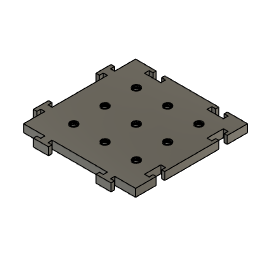
Threaded Optical Breadboard (Autodesk Fusion 360 design; units mm, degrees)
Autodesk Fusion 360 part; units mm, degrees
(part 1 of 2)
sketch "Sketch1" plane through (0, 0, 0) normal (0, 0, 1) x (1, 0, 0) in component "Breadboard"
  line L0 (20.188, 20.188) -> (-20.188, 20.188) construction
  line L1 (-20.188, 20.188) -> (-20.188, -20.188) construction
  line L2 (-20.188, -20.188) -> (20.188, -20.188) construction
  line L3 (20.188, -20.188) -> (20.188, 20.188) construction
  line L4 (20.188, 20.188) -> (-20.188, -20.188) construction
  line L5 (-20.188, 20.188) -> (20.188, -20.188) construction
  line L6 (-20.188, 20.188) -> (20.188, 20.188) construction
  line L7 (20.188, 20.188) -> (20.188, 60.564) construction
  line L8 (20.188, 60.564) -> (-20.188, 60.564) construction
  line L9 (-20.188, 60.564) -> (-20.188, 20.188) construction
  line L10 (20.188, 60.564) -> (60.564, 60.564) construction
  line L11 (60.564, 60.564) -> (60.564, 20.188) construction
  line L12 (60.564, 20.188) -> (20.188, 20.188) construction
  line L13 (20.188, 20.188) -> (20.188, 60.564) construction
  line L14 (60.564, 20.188) -> (20.188, 20.188) construction
  line L15 (20.188, 20.188) -> (20.188, -20.188) construction
  line L16 (20.188, -20.188) -> (60.564, -20.188) construction
  line L17 (60.564, -20.188) -> (60.564, 20.188) construction
  line L18 (-20.188, -20.188) -> (20.188, -20.188) construction
  line L19 (20.188, -20.188) -> (20.188, -60.564) construction
  line L20 (20.188, -60.564) -> (-20.188, -60.564) construction
  line L21 (-20.188, -60.564) -> (-20.188, -20.188) construction
  line L22 (20.188, -20.188) -> (60.564, -20.188) construction
  line L23 (60.564, -20.188) -> (60.564, -60.564) construction
  line L24 (60.564, -60.564) -> (20.188, -60.564) construction
  line L25 (20.188, -60.564) -> (20.188, -20.188) construction
  line L26 (-20.188, 20.188) -> (-60.564, 20.188) construction
  line L27 (-60.564, 20.188) -> (-60.564, 60.564) construction
  line L28 (-60.564, 60.564) -> (-20.188, 60.564) construction
  line L29 (-20.188, 60.564) -> (-20.188, 20.188) construction
  line L30 (-60.564, 20.188) -> (-20.188, 20.188) construction
  line L31 (-20.188, 20.188) -> (-20.188, -20.188) construction
  line L32 (-20.188, -20.188) -> (-60.564, -20.188) construction
  line L33 (-60.564, -20.188) -> (-60.564, 20.188) construction
  line L34 (-60.564, -20.188) -> (-20.188, -20.188) construction
  line L35 (-20.188, -20.188) -> (-20.188, -60.564) construction
  line L36 (-20.188, -60.564) -> (-60.564, -60.564) construction
  line L37 (-60.564, -60.564) -> (-60.564, -20.188) construction
  line L38 (72.5, 72.5) -> (-72.5, 72.5)
  line L39 (-72.5, 72.5) -> (-72.5, -72.5)
  line L40 (-72.5, -72.5) -> (72.5, -72.5)
  line L41 (72.5, -72.5) -> (72.5, 72.5)
  line L42 (72.5, 72.5) -> (-72.5, -72.5) construction
  line L43 (-72.5, 72.5) -> (72.5, -72.5) construction
  circle A0 centre (-40.376, 40.376) radius 5
  circle A1 centre (0, 40.376) radius 5
  circle A2 centre (40.376, 40.376) radius 5
  circle A3 centre (40.376, 0) radius 5
  circle A4 centre (0, 0) radius 5
  circle A5 centre (40.376, -40.376) radius 5
  circle A6 centre (0, -40.376) radius 5
  circle A7 centre (-40.376, -40.376) radius 5
  circle A8 centre (-40.376, 0) radius 5
  line L44 (-60.564, 60.564) -> (-60.564, 72.5) construction
  line L45 (-20.188, 60.564) -> (-20.188, 72.5) construction
  line L46 (20.188, 60.564) -> (20.188, 72.5) construction
  line L47 (60.564, 60.564) -> (60.564, 72.5) construction
  line L48 (60.564, 60.564) -> (72.5, 60.564) construction
  line L49 (60.564, 20.188) -> (72.5, 20.188) construction
  line L50 (60.564, -20.188) -> (72.5, -20.188) construction
  line L51 (60.564, -60.564) -> (72.5, -60.564) construction
  line L52 (60.564, -60.564) -> (60.564, -72.5) construction
  line L53 (20.188, -60.564) -> (20.188, -72.5) construction
  line L54 (-20.188, -60.564) -> (-20.188, -72.5) construction
  line L55 (-60.564, -60.564) -> (-60.564, -72.5) construction
  line L56 (-60.564, -60.564) -> (-72.5, -60.564) construction
  line L57 (-60.564, -20.188) -> (-72.5, -20.188) construction
  line L58 (-60.564, 20.188) -> (-72.5, 20.188) construction
  line L59 (-60.564, 60.564) -> (-72.5, 60.564) construction
  line L60 (-40.376, 60.564) -> (-40.376, 72.5) construction
  line L61 (40.376, 60.564) -> (40.376, 72.5) construction
  line L62 (60.564, 40.376) -> (72.5, 40.376) construction
  line L63 (60.564, -40.376) -> (72.5, -40.376) construction
  line L64 (40.376, -60.564) -> (40.376, -72.5) construction
  line L65 (-40.376, -60.564) -> (-40.376, -72.5) construction
  line L66 (-60.564, -40.376) -> (-72.5, -40.376) construction
  line L67 (-60.564, 40.376) -> (-72.5, 40.376) construction
  line L68 (-40.376, 72.5) -> (-45.376, 72.5) construction
  line L69 (-40.376, 72.5) -> (-35.376, 72.5) construction
  line L70 (-45.376, 72.5) -> (-35.376, 72.5)
  line L71 (-35.376, 72.5) -> (-35.376, 67.5)
  line L72 (-35.376, 67.5) -> (-45.376, 67.5)
  line L73 (-45.376, 67.5) -> (-45.376, 72.5)
  line L74 (-35.376, 67.5) -> (-30.376, 67.5)
  line L75 (-30.376, 67.5) -> (-30.376, 62.5)
  line L76 (-30.376, 62.5) -> (-35.376, 62.5)
  line L77 (-35.376, 62.5) -> (-35.376, 67.5)
  line L78 (-35.376, 62.5) -> (-45.376, 62.5)
  line L79 (-45.376, 62.5) -> (-45.376, 67.5)
  line L80 (-45.376, 67.5) -> (-35.376, 67.5)
  line L81 (-35.376, 67.5) -> (-35.376, 62.5)
  line L82 (-45.376, 67.5) -> (-50.376, 67.5)
  line L83 (-50.376, 67.5) -> (-50.376, 62.5)
  line L84 (-50.376, 62.5) -> (-45.376, 62.5)
  line L85 (-45.376, 62.5) -> (-45.376, 67.5)
  line L86 (40.376, 72.5) -> (35.376, 72.5) construction
  line L87 (40.376, 72.5) -> (45.376, 72.5) construction
  line L88 (35.376, 72.5) -> (45.376, 72.5)
  line L89 (45.376, 72.5) -> (45.376, 67.5)
  line L90 (45.376, 67.5) -> (35.376, 67.5)
  line L91 (35.376, 67.5) -> (35.376, 72.5)
  line L92 (35.376, 67.5) -> (45.376, 67.5)
  line L93 (45.376, 67.5) -> (45.376, 62.5)
  line L94 (45.376, 62.5) -> (35.376, 62.5)
  line L95 (35.376, 62.5) -> (35.376, 67.5)
  line L96 (45.376, 62.5) -> (50.376, 62.5)
  line L97 (50.376, 62.5) -> (50.376, 67.5)
  line L98 (50.376, 67.5) -> (45.376, 67.5)
  line L99 (45.376, 67.5) -> (45.376, 62.5)
  line L100 (35.376, 62.5) -> (30.376, 62.5)
  line L101 (30.376, 62.5) -> (30.376, 67.5)
  line L102 (30.376, 67.5) -> (35.376, 67.5)
  line L103 (35.376, 67.5) -> (35.376, 62.5)
  line L104 (72.5, 40.376) -> (72.5, 45.376) construction
  line L105 (72.5, 40.376) -> (72.5, 35.376) construction
  line L106 (72.5, 45.376) -> (67.5, 45.376)
  line L107 (67.5, 45.376) -> (67.5, 35.376)
  line L108 (67.5, 35.376) -> (72.5, 35.376)
  line L109 (72.5, 35.376) -> (72.5, 45.376)
  line L110 (67.5, 45.376) -> (62.5, 45.376)
  line L111 (62.5, 45.376) -> (62.5, 35.376)
  line L112 (62.5, 35.376) -> (67.5, 35.376)
  line L113 (67.5, 35.376) -> (67.5, 45.376)
  line L114 (67.5, 45.376) -> (62.5, 45.376)
  line L115 (62.5, 45.376) -> (62.5, 50.376)
  line L116 (62.5, 50.376) -> (67.5, 50.376)
  line L117 (67.5, 50.376) -> (67.5, 45.376)
  line L118 (67.5, 35.376) -> (62.5, 35.376)
  line L119 (62.5, 35.376) -> (62.5, 30.376)
  line L120 (62.5, 30.376) -> (67.5, 30.376)
  line L121 (67.5, 30.376) -> (67.5, 35.376)
  line L122 (72.5, -40.376) -> (72.5, -35.376) construction
  line L123 (72.5, -40.376) -> (72.5, -45.376) construction
  line L124 (72.5, -45.376) -> (67.5, -45.376)
  line L125 (67.5, -45.376) -> (67.5, -35.376)
  line L126 (67.5, -35.376) -> (72.5, -35.376)
  line L127 (72.5, -35.376) -> (72.5, -45.376)
  line L128 (67.5, -35.376) -> (62.5, -35.376)
  line L129 (62.5, -35.376) -> (62.5, -45.376)
  line L130 (62.5, -45.376) -> (67.5, -45.376)
  line L131 (67.5, -45.376) -> (67.5, -35.376)
  line L132 (67.5, -35.376) -> (62.5, -35.376)
  line L133 (62.5, -35.376) -> (62.5, -30.376)
  line L134 (62.5, -30.376) -> (67.5, -30.376)
  line L135 (67.5, -30.376) -> (67.5, -35.376)
  line L136 (67.5, -45.376) -> (62.5, -45.376)
  line L137 (62.5, -45.376) -> (62.5, -50.376)
  line L138 (62.5, -50.376) -> (67.5, -50.376)
  line L139 (67.5, -50.376) -> (67.5, -45.376)
  line L140 (40.376, -72.5) -> (45.376, -72.5)
  line L141 (40.376, -72.5) -> (35.376, -72.5)
  line L142 (-40.376, -72.5) -> (-35.376, -72.5)
  line L143 (-40.376, -72.5) -> (-45.376, -72.5)
  line L144 (-72.5, -40.376) -> (-72.5, -45.376)
  line L145 (-72.5, -40.376) -> (-72.5, -35.376)
  line L146 (-72.5, 40.376) -> (-72.5, 35.376)
  line L147 (-72.5, 40.376) -> (-72.5, 45.376)
  line L148 (-72.5, 45.376) -> (-77.5, 45.376)
  line L149 (-77.5, 45.376) -> (-77.5, 35.376)
  line L150 (-77.5, 35.376) -> (-72.5, 35.376)
  line L151 (-72.5, 35.376) -> (-72.5, 45.376)
  line L152 (-77.5, 35.376) -> (-82.5, 35.376)
  line L153 (-82.5, 35.376) -> (-82.5, 45.376)
  line L154 (-82.5, 45.376) -> (-77.5, 45.376)
  line L155 (-77.5, 45.376) -> (-77.5, 35.376)
  line L156 (-77.5, 35.376) -> (-82.5, 35.376)
  line L157 (-82.5, 35.376) -> (-82.5, 30.376)
  line L158 (-82.5, 30.376) -> (-77.5, 30.376)
  line L159 (-77.5, 30.376) -> (-77.5, 35.376)
  line L160 (-77.5, 45.376) -> (-82.5, 45.376)
  line L161 (-82.5, 45.376) -> (-82.5, 50.376)
  line L162 (-82.5, 50.376) -> (-77.5, 50.376)
  line L163 (-77.5, 50.376) -> (-77.5, 45.376)
  line L164 (-72.5, -35.376) -> (-77.5, -35.376)
  line L165 (-77.5, -35.376) -> (-77.5, -45.376)
  line L166 (-77.5, -45.376) -> (-72.5, -45.376)
  line L167 (-72.5, -45.376) -> (-72.5, -35.376)
  line L168 (-77.5, -45.376) -> (-82.5, -45.376)
  line L169 (-82.5, -45.376) -> (-82.5, -35.376)
  line L170 (-82.5, -35.376) -> (-77.5, -35.376)
  line L171 (-77.5, -35.376) -> (-77.5, -45.376)
  line L172 (-77.5, -35.376) -> (-82.5, -35.376)
  line L173 (-82.5, -35.376) -> (-82.5, -30.376)
  line L174 (-82.5, -30.376) -> (-77.5, -30.376)
  line L175 (-77.5, -30.376) -> (-77.5, -35.376)
  line L176 (-77.5, -45.376) -> (-82.5, -45.376)
  line L177 (-82.5, -45.376) -> (-82.5, -50.376)
  line L178 (-82.5, -50.376) -> (-77.5, -50.376)
  line L179 (-77.5, -50.376) -> (-77.5, -45.376)
  line L180 (-45.376, -72.5) -> (-35.376, -72.5)
  line L181 (-35.376, -72.5) -> (-35.376, -77.5)
  line L182 (-35.376, -77.5) -> (-45.376, -77.5)
  line L183 (-45.376, -77.5) -> (-45.376, -72.5)
  line L184 (-35.376, -77.5) -> (-45.376, -77.5)
  line L185 (-45.376, -77.5) -> (-45.376, -82.5)
  line L186 (-45.376, -82.5) -> (-35.376, -82.5)
  line L187 (-35.376, -82.5) -> (-35.376, -77.5)
  line L188 (-35.376, -82.5) -> (-30.376, -82.5)
  line L189 (-30.376, -82.5) -> (-30.376, -77.5)
  line L190 (-30.376, -77.5) -> (-35.376, -77.5)
  line L191 (-35.376, -77.5) -> (-35.376, -82.5)
  line L192 (-45.376, -82.5) -> (-50.376, -82.5)
  line L193 (-50.376, -82.5) -> (-50.376, -77.5)
  line L194 (-50.376, -77.5) -> (-45.376, -77.5)
  line L195 (-45.376, -77.5) -> (-45.376, -82.5)
  line L196 (45.376, -72.5) -> (35.376, -72.5)
  line L197 (35.376, -72.5) -> (35.376, -77.5)
  line L198 (35.376, -77.5) -> (45.376, -77.5)
  line L199 (45.376, -77.5) -> (45.376, -72.5)
  line L200 (35.376, -77.5) -> (45.376, -77.5)
  line L201 (45.376, -77.5) -> (45.376, -82.5)
  line L202 (45.376, -82.5) -> (35.376, -82.5)
  line L203 (35.376, -82.5) -> (35.376, -77.5)
  line L204 (45.376, -77.5) -> (50.376, -77.5)
  line L205 (50.376, -77.5) -> (50.376, -82.5)
  line L206 (50.376, -82.5) -> (45.376, -82.5)
  line L207 (45.376, -82.5) -> (45.376, -77.5)
  line L208 (35.376, -82.5) -> (30.376, -82.5)
  line L209 (30.376, -82.5) -> (30.376, -77.5)
  line L210 (30.376, -77.5) -> (35.376, -77.5)
  line L211 (35.376, -77.5) -> (35.376, -82.5)
  dimension "d3" = 40.376
  dimension "d4" = 40.376
  dimension "d5" = 40.376
  dimension "d6" = 40.376
  dimension "d7" = 40.376
  dimension "d8" = 40.376
  dimension "d9" = 40.376
  dimension "d10" = 40.376
  dimension "d11" = 145
  dimension "d12" = 145
  dimension "d13" = 10
  dimension "d14" = 10
  dimension "d15" = 10
  dimension "d16" = 10
  dimension "d17" = 10
  dimension "d18" = 10
  dimension "d19" = 10
  dimension "d20" = 10
  dimension "d21" = 10
  dimension "d22" = 5
  dimension "d23" = 5
  dimension "d24" = 10
  dimension "d25" = 5
  dimension "d26" = 5
  dimension "d27" = 5
  dimension "d28" = 5
  dimension "d29" = 5
  dimension "d30" = 5
  dimension "d31" = 5
  dimension "d32" = 5
  dimension "d33" = 5
  dimension "d34" = 5
  dimension "d35" = 5
  dimension "d36" = 5
  dimension "d37" = 5
  dimension "d38" = 5
  dimension "d39" = 5
  dimension "d40" = 5
  dimension "d41" = 5
  dimension "d42" = 5
  dimension "d43" = 5
  dimension "d44" = 5
  dimension "d45" = 5
  dimension "d46" = 5
  dimension "d47" = 5
  dimension "d48" = 5
  dimension "d49" = 5
  dimension "d50" = 5
  dimension "d51" = 5
  dimension "d52" = 5
  dimension "d53" = 5
  dimension "d54" = 5
  dimension "d55" = 5
  dimension "d56" = 5
  dimension "d57" = 5
  dimension "d58" = 5
  dimension "d59" = 5
  dimension "d60" = 5
  dimension "d61" = 5
  dimension "d62" = 5
  dimension "d63" = 5
  dimension "d64" = 5
  dimension "d65" = 5
  dimension "d66" = 5
  dimension "d67" = 10
  dimension "d68" = 5
  dimension "d69" = 5
  dimension "d70" = 5
  constraint coincident A4.centre origin
  constraint horizontal L0
  constraint perpendicular L0 L1
  constraint parallel L0 L2
  constraint parallel L1 L3
  constraint coincident L4 A4.centre
  constraint coincident L5 A4.centre
  constraint horizontal L6
  constraint vertical L7
  constraint horizontal L8
  constraint vertical L9
  constraint horizontal L10
  constraint vertical L11
  constraint horizontal L12
  constraint vertical L13
  constraint horizontal L14
  constraint vertical L15
  constraint horizontal L16
  constraint vertical L17
  constraint horizontal L18
  constraint vertical L19
  constraint horizontal L20
  constraint vertical L21
  constraint horizontal L22
  constraint vertical L23
  constraint horizontal L24
  constraint vertical L25
  constraint horizontal L26
  constraint vertical L27
  constraint horizontal L28
  constraint vertical L29
  constraint horizontal L30
  constraint vertical L31
  constraint horizontal L32
  constraint vertical L33
  constraint horizontal L34
  constraint vertical L35
  constraint horizontal L36
  constraint vertical L37
  constraint horizontal L38
  constraint perpendicular L38 L39
  constraint parallel L38 L40
  constraint parallel L39 L41
  constraint coincident L42 A4.centre
  constraint coincident L43 A4.centre
  constraint coincident L43 A0.centre
  constraint coincident L42 A2.centre
  constraint coincident L43 A5.centre
  constraint coincident L42 A7.centre
  constraint coincident L38 L44.end
  constraint perpendicular L38 L44
  constraint coincident L38 L45.end
  constraint perpendicular L38 L45
  constraint coincident L38 L46.end
  constraint perpendicular L38 L46
  constraint coincident L38 L47.end
  constraint perpendicular L38 L47
  constraint coincident L41 L48.end
  constraint perpendicular L41 L48
  constraint coincident L41 L49.end
  constraint perpendicular L41 L49
  constraint coincident L41 L50.end
  constraint perpendicular L41 L50
  constraint coincident L41 L51.end
  constraint perpendicular L41 L51
  constraint coincident L40 L52.end
  constraint perpendicular L40 L52
  constraint coincident L40 L53.end
  constraint perpendicular L40 L53
  constraint coincident L40 L54.end
  constraint perpendicular L40 L54
  constraint coincident L40 L55.end
  constraint perpendicular L40 L55
  constraint coincident L39 L56.end
  constraint perpendicular L39 L56
  constraint coincident L39 L57.end
  constraint perpendicular L39 L57
  constraint perpendicular L33 L58
  constraint coincident L39 L59.end
  constraint perpendicular L39 L59
  constraint midpoint L28 L60.start
  constraint coincident L38 L60.end
  constraint perpendicular L38 L60
  constraint midpoint L10 L61.start
  constraint coincident L38 L61.end
  constraint perpendicular L38 L61
  constraint midpoint L11 L62.start
  constraint coincident L41 L62.end
  constraint perpendicular L41 L62
  constraint midpoint L23 L63.start
  constraint coincident L41 L63.end
  constraint perpendicular L41 L63
  constraint midpoint L24 L64.start
  constraint coincident L40 L64.end
  constraint perpendicular L40 L64
  constraint midpoint L36 L65.start
  constraint coincident L40 L65.end
  constraint perpendicular L40 L65
  constraint midpoint L37 L66.start
  constraint coincident L39 L66.end
  constraint perpendicular L39 L66
  constraint midpoint L27 L67.start
  constraint coincident L39 L67.end
  constraint perpendicular L39 L67
  constraint perpendicular L60 L68
  constraint coincident L38 L69.end
  constraint horizontal L70
  constraint vertical L71
  constraint horizontal L72
  constraint vertical L73
  constraint horizontal L74
  constraint vertical L75
  constraint horizontal L76
  constraint vertical L77
  constraint horizontal L78
  constraint vertical L79
  constraint horizontal L80
  constraint vertical L81
  constraint horizontal L82
  constraint vertical L83
  constraint horizontal L84
  constraint vertical L85
  constraint coincident L38 L86.end
  constraint perpendicular L61 L87
  constraint horizontal L88
  constraint vertical L89
  constraint horizontal L90
  constraint vertical L91
  constraint horizontal L92
  constraint vertical L93
  constraint horizontal L94
  constraint vertical L95
  constraint horizontal L96
  constraint vertical L97
  constraint horizontal L98
  constraint vertical L99
  constraint horizontal L100
  constraint vertical L101
  constraint horizontal L102
  constraint vertical L103
  constraint perpendicular L62 L104
  constraint perpendicular L62 L105
  constraint horizontal L106
  constraint vertical L107
  constraint horizontal L108
  constraint vertical L109
  constraint horizontal L110
  constraint vertical L111
  constraint horizontal L112
  constraint vertical L113
  constraint horizontal L114
  constraint vertical L115
  constraint horizontal L116
  constraint vertical L117
  constraint horizontal L118
  constraint vertical L119
  constraint horizontal L120
  constraint vertical L121
  constraint perpendicular L63 L122
  constraint perpendicular L63 L123
  constraint horizontal L124
  constraint vertical L125
  constraint horizontal L126
  constraint vertical L127
  constraint horizontal L128
  constraint vertical L129
  constraint horizontal L130
  constraint vertical L131
  constraint horizontal L132
  constraint vertical L133
  constraint horizontal L134
  constraint vertical L135
  constraint horizontal L136
  constraint vertical L137
  constraint horizontal L138
  constraint vertical L139
  constraint coincident L40 L140.end
  constraint perpendicular L64 L141
  constraint perpendicular L65 L142
  constraint perpendicular L65 L143
  constraint perpendicular L66 L144
  constraint perpendicular L66 L145
  constraint perpendicular L67 L146
  constraint perpendicular L67 L147
  constraint horizontal L148
  constraint vertical L149
  constraint horizontal L150
  constraint vertical L151
  constraint horizontal L152
  constraint vertical L153
  constraint horizontal L154
  constraint vertical L155
  constraint horizontal L156
  constraint vertical L157
  constraint horizontal L158
  constraint vertical L159
  constraint horizontal L160
  constraint vertical L161
  constraint horizontal L162
  constraint vertical L163
  constraint horizontal L164
  constraint vertical L165
  constraint horizontal L166
  constraint vertical L167
  constraint horizontal L168
  constraint vertical L169
  constraint horizontal L170
  constraint vertical L171
  constraint horizontal L172
  constraint vertical L173
  constraint horizontal L174
  constraint vertical L175
  constraint horizontal L176
  constraint vertical L177
  constraint horizontal L178
  constraint vertical L179
  constraint horizontal L180
  constraint vertical L181
  constraint horizontal L182
  constraint vertical L183
  constraint horizontal L184
  constraint vertical L185
  constraint horizontal L186
  constraint vertical L187
  constraint horizontal L188
  constraint vertical L189
  constraint horizontal L190
  constraint vertical L191
  constraint horizontal L192
  constraint vertical L193
  constraint horizontal L194
  constraint vertical L195
  constraint horizontal L196
  constraint vertical L197
  constraint horizontal L198
  constraint vertical L199
  constraint horizontal L200
  constraint vertical L201
  constraint horizontal L202
  constraint vertical L203
  constraint horizontal L204
  constraint vertical L205
  constraint horizontal L206
  constraint vertical L207
  constraint horizontal L208
  constraint vertical L209
  constraint horizontal L210
  constraint vertical L211
  measures "d3" distance of L1.end L2.end
  measures "d4" distance of L0.end L1.end
  measures "d5" distance of L0.end L8.end
  measures "d6" distance of L7.end L10.end
  measures "d7" distance of L7.end L0.start
  measures "d8" distance of L1.end L20.end
  measures "d9" distance of L0.end L26.end
  measures "d10" distance of L0.end L8.end
  measures "d11" distance of L39.end L40.end
  measures "d12" distance of L38.end L39.end
  measures "d13" diameter of A0
  measures "d14" diameter of A1
  measures "d15" diameter of A2
  measures "d16" diameter of A3
  measures "d17" diameter of A4
  measures "d18" diameter of A5
  measures "d19" diameter of A6
  measures "d20" diameter of A7
  measures "d21" diameter of A8
  measures "d22" distance of L60.end L68.end
  measures "d23" distance of L60.end L69.end
  measures "d24" distance of L68.end L69.end
  measures "d25" distance of L68.end L72.end
  measures "d26" distance of L71.end L74.end
  measures "d27" distance of L71.end L76.end
  measures "d28" distance of L72.end L82.end
  measures "d29" distance of L61.end L86.end
  measures "d30" distance of L61.end L87.end
  measures "d31" distance of L86.end L90.end
  measures "d32" distance of L90.end L94.end
  measures "d33" distance of L93.end L96.end
  measures "d34" distance of L94.end L100.end
  measures "d35" distance of L62.end L104.end
  measures "d36" distance of L62.end L105.end
  measures "d37" distance of L104.end L106.end
  measures "d38" distance of L106.end L110.end
  measures "d39" distance of L106.end L116.end
  measures "d40" distance of L107.end L120.end
  measures "d41" distance of L63.end L122.end
  measures "d42" distance of L63.end L123.end
  measures "d43" distance of L123.end L124.end
  measures "d44" distance of L125.end L128.end
  measures "d45" distance of L125.end L134.end
  measures "d46" distance of L124.end L138.end
  measures "d47" distance of L64.end L140.end
  measures "d48" distance of L64.end L141.end
  measures "d49" distance of L65.end L142.end
  measures "d50" distance of L65.end L143.end
  measures "d51" distance of L66.end L144.end
  measures "d52" distance of L66.end L145.end
  measures "d53" distance of L67.end L146.end
  measures "d54" distance of L67.end L147.end
  measures "d55" distance of L147.end L148.end
  measures "d56" distance of L149.end L152.end
  measures "d57" distance of L149.end L158.end
  measures "d58" distance of L148.end L162.end
  measures "d59" distance of L165.end L168.end
  measures "d60" distance of L164.end L174.end
  measures "d61" distance of L165.end L168.end
  measures "d62" distance of L165.end L178.end
  measures "d63" distance of L143.end L182.end
  measures "d64" distance of L181.end L186.end
  measures "d65" distance of L186.end L188.end
  measures "d66" distance of L185.end L192.end
  measures "d67" distance of L197.end L198.end
  measures "d68" distance of L197.end L202.end
  measures "d69" distance of L198.end L204.end
  measures "d70" distance of L202.end L208.end
extrude "Extrude1" add sketch "Sketch1" along normal blind 10 contours L38 L39 L40 L41 L71 L73 L74 L75 L76 L78 L82 L83 L84 L89 L91 L94 L96 L97 L98 L100 L101 L102 L106 L108 L111 L115 L116 L117 L119 L120 L121 L124 L126 L129 L133 L134 L135 L137 L138 L139 L140 L141 L142 L143 L144 L145 L146 L147 L151 L167 L180 L196 | L39 L146 L147 L148 L149 L150 L151 L155 | L40 L140 L141 L196 L197 L198 L199 L200 | L149 L152 L153 L154 L155 L156 L160 | L154 L160 L161 L162 L163 | L198 L200 L201 L202 L203 L207 L211 | L201 L204 L205 L206 L207 | L152 L156 L157 L158 L159 | L203 L208 L209 L210 L211 | L39 L144 L145 L164 L165 L166 L167 L171 | L40 L142 L143 L180 L181 L182 L183 L184 | L165 L168 L169 L170 L171 L172 L176 | L170 L172 L173 L174 L175 | L182 L184 L185 L186 L187 L191 L195 | L187 L188 L189 L190 L191 | L168 L176 L177 L178 L179 | L185 L192 L193 L194 L195 makes body 1 in component "Breadboard"
extrude "Extrude2" cut 3 faces at (-82.5, 47.0427, 3.3333) (-82.5, 38.7093, 3.3333) (-82.5, 33.7093, 3.3333) along direction (1, 0, 0) blind 0.25 on bodies 1 bodies 1 in component "Breadboard"
extrude "Extrude3" cut 1 faces at (-80.6667, 30.376, 3.3333) along direction (0, 1, 0) blind 0.25 on bodies 1 bodies 1 in component "Breadboard"
extrude "Extrude4" cut 1 faces at (-80.6667, 50.376, 3.3333) along direction (0, -1, 0) blind 0.25 on bodies 1 bodies 1 in component "Breadboard"
extrude "Extrude5" cut 2 faces at (-77.5, 48.5427, 3.3333) (-77.5, 32.2093, 3.3333) along direction (-1, 0, 0) blind 0.25 on bodies 1 bodies 1 in component "Breadboard"
extrude "Extrude6" cut 1 faces at (-74.25, 45.376, 3.3333) along direction (0, -1, 0) blind 0.25 on bodies 1 bodies 1 in component "Breadboard"
extrude "Extrude7" cut 1 faces at (-76, 35.376, 3.3333) along direction (0, 1, 0) blind 0.25 on bodies 1 bodies 1 in component "Breadboard"
extrude "Extrude8" cut 1 faces at (-82.5, -37.0427, 3.3333) along direction (1, 0, 0) blind 0.25 on bodies 1 bodies 1 in component "Breadboard"
extrude "Extrude9" cut 1 faces at (-80.6667, -50.376, 3.3333) along direction (0, 1, 0) blind 0.25 on bodies 1 bodies 1 in component "Breadboard"
extrude "Extrude10" cut 1 faces at (-80.6667, -30.376, 3.3333) along direction (0, -1, 0) blind 0.25 on bodies 1 bodies 1 in component "Breadboard"
extrude "Extrude11" cut 2 faces at (-77.5, -32.2093, 3.3333) (-77.5, -48.5427, 3.3333) along direction (-1, 0, 0) blind 0.25 on bodies 1 bodies 1 in component "Breadboard"
extrude "Extrude12" cut 1 faces at (-74.25, -35.376, 3.3333) along direction (0, -1, 0) blind 0.25 on bodies 1 bodies 1 in component "Breadboard"
extrude "Extrude13" cut 1 faces at (-76, -45.376, 3.3333) along direction (0, 1, 0) blind 0.25 on bodies 1 bodies 1 in component "Breadboard"
extrude "Extrude14" cut 2 faces at (-43.7093, -82.5, 3.3333) (43.7093, -82.5, 3.3333) along direction (0, 1, 0) blind 0.25 on bodies 1 bodies 1 in component "Breadboard"
extrude "Extrude15" cut 1 faces at (-30.376, -80.6667, 3.3333) along direction (-1, 0, 0) blind 0.25 on bodies 1 bodies 1 in component "Breadboard"
extrude "Extrude16" cut 1 faces at (-50.376, -80.6667, 3.3333) along direction (1, 0, 0) blind 0.25 on bodies 1 bodies 1 in component "Breadboard"
extrude "Extrude17" cut 2 faces at (-48.5427, -77.5, 3.3333) (-32.2093, -77.5, 3.3333) along direction (0, -1, 0) blind 0.25 on bodies 1 bodies 1 in component "Breadboard"
extrude "Extrude18" cut 1 faces at (-45.376, -74.25, 3.3333) along direction (1, 0, 0) blind 0.25 on bodies 1 bodies 1 in component "Breadboard"
extrude "Extrude19" cut 1 faces at (-35.376, -74.25, 3.3333) along direction (-1, 0, 0) blind 0.25 on bodies 1 bodies 1 in component "Breadboard"
extrude "Extrude20" cut 2 faces at (47.0427, -77.5, 3.3333) (32.0427, -77.5, 6.6667) along direction (0, -1, 0) blind 0.25 on bodies 1 bodies 1 in component "Breadboard"
extrude "Extrude21" cut 1 faces at (50.376, -79.25, 3.3333) along direction (-1, 0, 0) blind 0.25 on bodies 1 bodies 1 in component "Breadboard"
extrude "Extrude22" cut 1 faces at (30.376, -80.75, 3.3333) along direction (1, 0, 0) blind 0.25 on bodies 1 bodies 1 in component "Breadboard"
extrude "Extrude23" cut 1 faces at (35.376, -74.25, 3.3333) along direction (1, 0, 0) blind 0.25 on bodies 1 bodies 1 in component "Breadboard"
extrude "Extrude24" cut 1 faces at (45.376, -76, 3.3333) along direction (-1, 0, 0) blind 0.25 on bodies 1 bodies 1 in component "Breadboard"
sketch "Sketch2" plane through (0, 0, 10) normal (0, 0, 1) x (-1, 0, 0) in component "Breadboard"
  line L0 (-45.126, 72.5) -> (-72.5, 72.5)
  line L1 (-72.5, 72.5) -> (-72.5, 45.376)
  line L2 (-72.5, 45.376) -> (-67.5, 45.376)
  line L3 (-67.5, 45.376) -> (-67.5, 50.376)
  line L4 (-67.5, 50.376) -> (-62.5, 50.376)
  line L5 (-62.5, 50.376) -> (-62.5, 30.376)
  line L6 (-62.5, 30.376) -> (-67.5, 30.376)
  line L7 (-67.5, 30.376) -> (-67.5, 35.376)
  line L8 (-67.5, 35.376) -> (-72.5, 35.376)
  line L9 (-72.5, 35.376) -> (-72.5, -35.376)
  line L10 (-72.5, -35.376) -> (-67.5, -35.376)
  line L11 (-67.5, -35.376) -> (-67.5, -30.376)
  line L12 (-67.5, -30.376) -> (-62.5, -30.376)
  line L13 (-62.5, -30.376) -> (-62.5, -50.376)
  line L14 (-62.5, -50.376) -> (-67.5, -50.376)
  line L15 (-67.5, -50.376) -> (-67.5, -45.376)
  line L16 (-67.5, -45.376) -> (-72.5, -45.376)
  line L17 (-72.5, -45.376) -> (-72.5, -72.5)
  line L18 (-72.5, -72.5) -> (-45.376, -72.5)
  line L19 (-45.376, -72.5) -> (-45.376, -67.5)
  line L20 (-45.376, -67.5) -> (-50.376, -67.5)
  line L21 (-50.376, -67.5) -> (-50.376, -62.5)
  line L22 (-50.376, -62.5) -> (-30.376, -62.5)
  line L23 (-30.376, -62.5) -> (-30.376, -67.5)
  line L24 (-30.376, -67.5) -> (-35.376, -67.5)
  line L25 (-35.376, -67.5) -> (-35.376, -72.5)
  line L26 (-35.376, -72.5) -> (35.376, -72.5)
  line L27 (35.376, -72.5) -> (35.376, -67.5)
  line L28 (35.376, -67.5) -> (30.376, -67.5)
  line L29 (30.376, -67.5) -> (30.376, -62.5)
  line L30 (30.376, -62.5) -> (50.376, -62.5)
  line L31 (50.376, -62.5) -> (50.376, -67.5)
  line L32 (50.376, -67.5) -> (45.376, -67.5)
  line L33 (45.376, -67.5) -> (45.376, -72.5)
  line L34 (45.376, -72.5) -> (72.5, -72.5)
  line L35 (72.5, -72.5) -> (72.5, -45.126)
  line L36 (72.5, -45.126) -> (77.75, -45.126)
  line L37 (77.75, -45.126) -> (77.75, -50.126)
  line L38 (77.75, -50.126) -> (82.25, -50.126)
  line L39 (82.25, -50.126) -> (82.25, -30.626)
  line L40 (82.25, -30.626) -> (77.75, -30.626)
  line L41 (77.75, -30.626) -> (77.75, -35.626)
  line L42 (77.75, -35.626) -> (72.5, -35.626)
  line L43 (72.5, -35.626) -> (72.5, 35.626)
  line L44 (72.5, 35.626) -> (77.75, 35.626)
  line L45 (77.75, 35.626) -> (77.75, 30.626)
  line L46 (77.75, 30.626) -> (82.25, 30.626)
  line L47 (82.25, 30.626) -> (82.25, 50.126)
  line L48 (82.25, 50.126) -> (77.75, 50.126)
  line L49 (77.75, 50.126) -> (77.75, 45.126)
  line L50 (77.75, 45.126) -> (72.5, 45.126)
  line L51 (72.5, 45.126) -> (72.5, 72.5)
  line L52 (72.5, 72.5) -> (45.126, 72.5)
  line L53 (45.126, 72.5) -> (45.126, 77.75)
  line L54 (45.126, 77.75) -> (50.126, 77.75)
  line L55 (50.126, 77.75) -> (50.126, 82.25)
  line L56 (50.126, 82.25) -> (30.626, 82.25)
  line L57 (30.626, 82.25) -> (30.626, 77.75)
  line L58 (30.626, 77.75) -> (35.626, 77.75)
  line L59 (35.626, 77.75) -> (35.626, 72.5)
  line L60 (35.626, 72.5) -> (-35.626, 72.5)
  line L61 (-35.626, 72.5) -> (-35.626, 77.75)
  line L62 (-35.626, 77.75) -> (-30.626, 77.75)
  line L63 (-30.626, 77.75) -> (-30.626, 82.25)
  line L64 (-30.626, 82.25) -> (-50.126, 82.25)
  line L65 (-50.126, 82.25) -> (-50.126, 77.75)
  line L66 (-50.126, 77.75) -> (-45.126, 77.75)
  line L67 (-45.126, 77.75) -> (-45.126, 72.5)
  circle A0 centre (40.376, 0) radius 5
  circle A1 centre (40.376, 40.376) radius 5
  circle A2 centre (0, 40.376) radius 5
  circle A3 centre (-40.376, 40.376) radius 5
  circle A4 centre (0, 0) radius 5
  circle A5 centre (-40.376, 0) radius 5
  circle A6 centre (-40.376, -40.376) radius 5
  circle A7 centre (0, -40.376) radius 5
  circle A8 centre (40.376, -40.376) radius 5
  line L68 (50.376, -62.5) -> (30.376, -62.5)
  line L69 (30.376, -62.5) -> (30.376, -67.5)
  line L70 (30.376, -67.5) -> (50.376, -67.5)
  line L71 (50.376, -67.5) -> (50.376, -62.5)
  line L72 (35.376, -67.5) -> (45.376, -67.5)
  line L73 (45.376, -67.5) -> (45.376, -72.5)
  line L74 (45.376, -72.5) -> (35.376, -72.5)
  line L75 (35.376, -72.5) -> (35.376, -67.5)
  line L76 (45.376, -72.5) -> (55.376, -72.5)
  line L77 (55.376, -72.5) -> (25.376, -72.5)
  line L78 (25.376, -72.5) -> (25.376, -57.5)
  line L79 (25.376, -57.5) -> (55.376, -57.5)
  line L80 (55.376, -57.5) -> (55.376, -72.5)
  dimension "d119" = 10
  dimension "d120" = 30
  dimension "d121" = 15
  constraint horizontal L68
  constraint vertical L69
  constraint horizontal L70
  constraint vertical L71
  constraint coincident L28.end L29.start
  constraint coincident L30.end L31.start
  constraint horizontal L72
  constraint vertical L73
  constraint horizontal L74
  constraint vertical L75
  constraint coincident L33.end L34.start
  constraint coincident L27.end L28.start
  constraint perpendicular L73 L76
  constraint horizontal L77
  constraint vertical L78
  constraint horizontal L79
  constraint vertical L80
  measures "d119" distance of L33.end L76.end
  measures "d120" distance of L76.end L77.end
  measures "d121" distance of L76.end L79.end
extrude "Extrude25" add sketch "Sketch2" along normal blind 5 separate body contours L26 L27 L28 L29 L30 L31 L32 L33 L34 L68 L69 L70 L71 L73 L75 L76 L77 L78 L79 L80 makes body 2 in component "Breadboard"
extrude "Extrude26" cut 1 faces at (-37.0427, 62.5, 11.6667) along direction (0, -1, 0) blind 0.25 on bodies 2 bodies 2 in component "Breadboard"
extrude "Extrude27" cut 1 faces at (-30.376, 65.75, 11.6667) along direction (1, 0, 0) blind 0.25 on bodies 2 bodies 2 in component "Breadboard"
extrude "Extrude28" cut 1 faces at (-50.376, 64, 11.6667) along direction (-1, 0, 0) blind 0.25 on bodies 2 bodies 2 in component "Breadboard"
extrude "Extrude29" cut 2 faces at (-33.626, 67.5, 11.6667) (-48.876, 67.5, 11.6667) along direction (0, 1, 0) blind 0.25 on bodies 2 bodies 2 in component "Breadboard"
extrude "Extrude30" cut 1 faces at (-35.376, 70.9167, 11.6667) along direction (1, 0, 0) blind 0.25 on bodies 2 bodies 2 in component "Breadboard"
extrude "Extrude31" cut 1 faces at (-45.376, 69.3333, 11.6667) along direction (-1, 0, 0) blind 0.25 on bodies 2 bodies 2 in component "Breadboard"
extrude "Extrude32" cut 2 faces at (-28.626, 72.5, 11.6667) (-48.876, 72.5, 13.3333) along direction (0, -1, 0) blind 0.25 on bodies 2 bodies 2 in component "Breadboard"
copy_body "CutPasteBodies1" bodies 1 removing the originals makes body 3 in component "Breadboard"
copy_body "CutPasteBodies2" bodies 2 removing the originals makes body 4 in component "Breadboard"
extrude "Extrude1'" cut 1 faces at (-43.7927, 62.25, 11.6667) along direction (0, -1, 0) blind 0.25 on bodies 4 bodies 4 in component "Breadboard"
extrude "Extrude2'" cut 1 faces at (-30.126, 65.8333, 11.6667) along direction (1, 0, 0) blind 0.25 on bodies 4 bodies 4 in component "Breadboard"
extrude "Extrude3'" cut 1 faces at (-50.626, 63.9167, 11.6667) along direction (-1, 0, 0) blind 0.25 on bodies 4 bodies 4 in component "Breadboard"
extrude "Extrude4'" cut 2 faces at (-49.126, 67.75, 11.6667) (-33.376, 67.75, 11.6667) along direction (0, 1, 0) blind 0.25 on bodies 4 bodies 4 in component "Breadboard"
extrude "Extrude5'" cut 1 faces at (-45.626, 69.4167, 11.6667) along direction (-1, 0, 0) blind 0.25 on bodies 4 bodies 4 in component "Breadboard"
extrude "Extrude6'" cut 1 faces at (-35.126, 70.8333, 11.6667) along direction (1, 0, 0) blind 0.25 on bodies 4 bodies 4 in component "Breadboard"
extrude "Extrude7'" cut 2 faces at (-28.5427, 72.25, 11.6667) (-49.0427, 72.25, 13.3333) along direction (0, -1, 0) blind 0.25 on bodies 4 bodies 4 in component "Breadboard"
sketch "Sketch3" plane through (0, 0, 10) normal (0, 0, 1) x (-1, 0, 0) in component "Breadboard"
  line L0 (-45.126, 72.5) -> (-72.5, 72.5)
  line L1 (-72.5, 72.5) -> (-72.5, 45.376)
  line L2 (-72.5, 45.376) -> (-67.5, 45.376)
  line L3 (-67.5, 45.376) -> (-67.5, 50.376)
  line L4 (-67.5, 50.376) -> (-62.5, 50.376)
  line L5 (-62.5, 50.376) -> (-62.5, 30.376)
  line L6 (-62.5, 30.376) -> (-67.5, 30.376)
  line L7 (-67.5, 30.376) -> (-67.5, 35.376)
  line L8 (-67.5, 35.376) -> (-72.5, 35.376)
  line L9 (-72.5, 35.376) -> (-72.5, -35.376)
  line L10 (-72.5, -35.376) -> (-67.5, -35.376)
  line L11 (-67.5, -35.376) -> (-67.5, -30.376)
  line L12 (-67.5, -30.376) -> (-62.5, -30.376)
  line L13 (-62.5, -30.376) -> (-62.5, -50.376)
  line L14 (-62.5, -50.376) -> (-67.5, -50.376)
  line L15 (-67.5, -50.376) -> (-67.5, -45.376)
  line L16 (-67.5, -45.376) -> (-72.5, -45.376)
  line L17 (-72.5, -45.376) -> (-72.5, -72.5)
  line L18 (-72.5, -72.5) -> (-45.376, -72.5)
  line L19 (-45.376, -72.5) -> (-45.376, -67.5)
  line L20 (-45.376, -67.5) -> (-50.376, -67.5)
  line L21 (-50.376, -67.5) -> (-50.376, -62.5)
  line L22 (-50.376, -62.5) -> (-30.376, -62.5)
  line L23 (-30.376, -62.5) -> (-30.376, -67.5)
  line L24 (-30.376, -67.5) -> (-35.376, -67.5)
  line L25 (-35.376, -67.5) -> (-35.376, -72.5)
  line L26 (-35.376, -72.5) -> (35.376, -72.5)
  line L27 (35.376, -72.5) -> (35.376, -67.5)
  line L28 (35.376, -67.5) -> (30.376, -67.5)
  line L29 (30.376, -67.5) -> (30.376, -62.5)
  line L30 (30.376, -62.5) -> (50.376, -62.5)
  line L31 (50.376, -62.5) -> (50.376, -67.5)
  line L32 (50.376, -67.5) -> (45.376, -67.5)
  line L33 (45.376, -67.5) -> (45.376, -72.5)
  line L34 (45.376, -72.5) -> (72.5, -72.5)
  line L35 (72.5, -72.5) -> (72.5, -45.126)
  line L36 (72.5, -45.126) -> (77.75, -45.126)
  line L37 (77.75, -45.126) -> (77.75, -50.126)
  line L38 (77.75, -50.126) -> (82.25, -50.126)
  line L39 (82.25, -50.126) -> (82.25, -30.626)
  line L40 (82.25, -30.626) -> (77.75, -30.626)
  line L41 (77.75, -30.626) -> (77.75, -35.626)
  line L42 (77.75, -35.626) -> (72.5, -35.626)
  line L43 (72.5, -35.626) -> (72.5, 35.626)
  line L44 (72.5, 35.626) -> (77.75, 35.626)
  line L45 (77.75, 35.626) -> (77.75, 30.626)
  line L46 (77.75, 30.626) -> (82.25, 30.626)
  line L47 (82.25, 30.626) -> (82.25, 50.126)
  line L48 (82.25, 50.126) -> (77.75, 50.126)
  line L49 (77.75, 50.126) -> (77.75, 45.126)
  line L50 (77.75, 45.126) -> (72.5, 45.126)
  line L51 (72.5, 45.126) -> (72.5, 72.5)
  line L52 (72.5, 72.5) -> (45.126, 72.5)
  line L53 (45.126, 72.5) -> (45.126, 77.75)
  line L54 (45.126, 77.75) -> (50.126, 77.75)
  line L55 (50.126, 77.75) -> (50.126, 82.25)
  line L56 (50.126, 82.25) -> (30.626, 82.25)
  line L57 (30.626, 82.25) -> (30.626, 77.75)
  line L58 (30.626, 77.75) -> (35.626, 77.75)
  line L59 (35.626, 77.75) -> (35.626, 72.5)
  line L60 (35.626, 72.5) -> (-35.626, 72.5)
  line L61 (-35.626, 72.5) -> (-35.626, 77.75)
  line L62 (-35.626, 77.75) -> (-30.626, 77.75)
  line L63 (-30.626, 77.75) -> (-30.626, 82.25)
  line L64 (-30.626, 82.25) -> (-50.126, 82.25)
  line L65 (-50.126, 82.25) -> (-50.126, 77.75)
  line L66 (-50.126, 77.75) -> (-45.126, 77.75)
  line L67 (-45.126, 77.75) -> (-45.126, 72.5)
  circle A0 centre (40.376, 0) radius 5
  circle A1 centre (40.376, 40.376) radius 5
  circle A2 centre (0, 40.376) radius 5
  circle A3 centre (-40.376, 40.376) radius 5
  circle A4 centre (0, 0) radius 5
  circle A5 centre (-40.376, 0) radius 5
  circle A6 centre (-40.376, -40.376) radius 5
  circle A7 centre (0, -40.376) radius 5
  circle A8 centre (40.376, -40.376) radius 5
  circle A9 centre (0, 0) radius 5.25
  circle A10 centre (0, 0) radius 7.5
  dimension "d152" = 10.5
  dimension "d153" = 15
  constraint coincident A4.centre A9.centre
  measures "d152" diameter of A9
  measures "d153" diameter of A10
extrude "Extrude33" add sketch "Sketch3" along normal blind 5 separate body contours A10 makes body 5 in component "Breadboard"
copy_body "CutPasteBodies3" bodies 5 removing the originals makes body 6 in component "Breadboard"
sketch "Sketch4" plane through (0, 0, 10) normal (0, 0, 1) x (-1, 0, 0)
  line L0 (-45.126, 72.5) -> (-72.5, 72.5)
  line L1 (-72.5, 72.5) -> (-72.5, 45.376)
  line L2 (-72.5, 45.376) -> (-67.5, 45.376)
  line L3 (-67.5, 45.376) -> (-67.5, 50.376)
  line L4 (-67.5, 50.376) -> (-62.5, 50.376)
  line L5 (-62.5, 50.376) -> (-62.5, 30.376)
  line L6 (-62.5, 30.376) -> (-67.5, 30.376)
  line L7 (-67.5, 30.376) -> (-67.5, 35.376)
  line L8 (-67.5, 35.376) -> (-72.5, 35.376)
  line L9 (-72.5, 35.376) -> (-72.5, -35.376)
  line L10 (-72.5, -35.376) -> (-67.5, -35.376)
  line L11 (-67.5, -35.376) -> (-67.5, -30.376)
  line L12 (-67.5, -30.376) -> (-62.5, -30.376)
  line L13 (-62.5, -30.376) -> (-62.5, -50.376)
  line L14 (-62.5, -50.376) -> (-67.5, -50.376)
  line L15 (-67.5, -50.376) -> (-67.5, -45.376)
  line L16 (-67.5, -45.376) -> (-72.5, -45.376)
  line L17 (-72.5, -45.376) -> (-72.5, -72.5)
  line L18 (-72.5, -72.5) -> (-45.376, -72.5)
  line L19 (-45.376, -72.5) -> (-45.376, -67.5)
  line L20 (-45.376, -67.5) -> (-50.376, -67.5)
  line L21 (-50.376, -67.5) -> (-50.376, -62.5)
  line L22 (-50.376, -62.5) -> (-30.376, -62.5)
  line L23 (-30.376, -62.5) -> (-30.376, -67.5)
  line L24 (-30.376, -67.5) -> (-35.376, -67.5)
  line L25 (-35.376, -67.5) -> (-35.376, -72.5)
  line L26 (-35.376, -72.5) -> (35.376, -72.5)
  line L27 (35.376, -72.5) -> (35.376, -67.5)
  line L28 (35.376, -67.5) -> (30.376, -67.5)
  line L29 (30.376, -67.5) -> (30.376, -62.5)
  line L30 (30.376, -62.5) -> (50.376, -62.5)
  line L31 (50.376, -62.5) -> (50.376, -67.5)
  line L32 (50.376, -67.5) -> (45.376, -67.5)
  line L33 (45.376, -67.5) -> (45.376, -72.5)
  line L34 (45.376, -72.5) -> (72.5, -72.5)
  line L35 (72.5, -72.5) -> (72.5, -45.126)
  line L36 (72.5, -45.126) -> (77.75, -45.126)
  line L37 (77.75, -45.126) -> (77.75, -50.126)
  line L38 (77.75, -50.126) -> (82.25, -50.126)
  line L39 (82.25, -50.126) -> (82.25, -30.626)
  line L40 (82.25, -30.626) -> (77.75, -30.626)
  line L41 (77.75, -30.626) -> (77.75, -35.626)
  line L42 (77.75, -35.626) -> (72.5, -35.626)
  line L43 (72.5, -35.626) -> (72.5, 35.626)
  line L44 (72.5, 35.626) -> (77.75, 35.626)
  line L45 (77.75, 35.626) -> (77.75, 30.626)
  line L46 (77.75, 30.626) -> (82.25, 30.626)
  line L47 (82.25, 30.626) -> (82.25, 50.126)
  line L48 (82.25, 50.126) -> (77.75, 50.126)
  line L49 (77.75, 50.126) -> (77.75, 45.126)
  line L50 (77.75, 45.126) -> (72.5, 45.126)
  line L51 (72.5, 45.126) -> (72.5, 72.5)
  line L52 (72.5, 72.5) -> (45.126, 72.5)
  line L53 (45.126, 72.5) -> (45.126, 77.75)
  line L54 (45.126, 77.75) -> (50.126, 77.75)
  line L55 (50.126, 77.75) -> (50.126, 82.25)
  line L56 (50.126, 82.25) -> (30.626, 82.25)
  line L57 (30.626, 82.25) -> (30.626, 77.75)
  line L58 (30.626, 77.75) -> (35.626, 77.75)
  line L59 (35.626, 77.75) -> (35.626, 72.5)
  line L60 (35.626, 72.5) -> (-35.626, 72.5)
  line L61 (-35.626, 72.5) -> (-35.626, 77.75)
  line L62 (-35.626, 77.75) -> (-30.626, 77.75)
  line L63 (-30.626, 77.75) -> (-30.626, 82.25)
  line L64 (-30.626, 82.25) -> (-50.126, 82.25)
  line L65 (-50.126, 82.25) -> (-50.126, 77.75)
  line L66 (-50.126, 77.75) -> (-45.126, 77.75)
  line L67 (-45.126, 77.75) -> (-45.126, 72.5)
  circle A0 centre (0, 0) radius 5
  circle A1 centre (-40.376, 0) radius 5
  circle A2 centre (-40.376, -40.376) radius 5
  circle A3 centre (0, -40.376) radius 5
  circle A4 centre (40.376, 40.376) radius 5
  circle A5 centre (-40.376, 40.376) radius 5
  circle A6 centre (0, 40.376) radius 5
  circle A7 centre (40.376, -40.376) radius 5
  circle A8 centre (40.376, 0) radius 5
  circle A9 centre (40.376, -40.376) radius 5.25
  circle A10 centre (0, -40.376) radius 5.25
  circle A11 centre (-40.376, -40.376) radius 5.25
  circle A12 centre (-40.376, 0) radius 5.25
  circle A13 centre (0, 0) radius 5.25
  circle A14 centre (40.376, 0) radius 5.25
  circle A15 centre (40.376, 40.376) radius 5.25
  circle A16 centre (0, 40.376) radius 5.25
  circle A17 centre (-40.376, 40.376) radius 5.25
  dimension "d156" = 10.5
  dimension "d157" = 10.5
  dimension "d158" = 10.5
  dimension "d159" = 10.5
  dimension "d160" = 10.5
  dimension "d161" = 10.5
  dimension "d162" = 10.5
  dimension "d163" = 10.5
  dimension "d164" = 10.5
  constraint concentric A7 A9
  constraint concentric A3 A10
  constraint concentric A2 A11
  constraint concentric A1 A12
  constraint coincident A0.centre A13.centre
  constraint concentric A8 A14
  constraint concentric A4 A15
  constraint concentric A6 A16
  constraint concentric A5 A17
  measures "d156" diameter of A9
  measures "d157" diameter of A10
  measures "d158" diameter of A11
  measures "d159" diameter of A12
  measures "d160" diameter of A13
  measures "d161" diameter of A14
  measures "d162" diameter of A15
  measures "d163" diameter of A16
  measures "d164" diameter of A17
extrude "Extrude8'" cut sketch "Sketch4" against normal up to surface (10 mm away) contours A0 | A1 | A2 | A3 | A4 | A5 | A6 | A7 | A8 | A9 | A10 | A11 | A12 | A13 | A14 | A15 | A16 | A17 bodies 3 in component "Breadboard"
extrude "Extrude9'" cut 1 faces at (-30.376, 65.8333, 3.3333) along direction (1, 0, 0) blind 0.5 on bodies 3 bodies 3 in component "Breadboard"
extrude "Extrude10'" cut 1 faces at (-43.5427, 62.5, 3.3333) along direction (0, -1, 0) blind 0.5 on bodies 3 bodies 3 in component "Breadboard"
extrude "Extrude11'" cut 1 faces at (-50.376, 65.6667, 6.6667) along direction (-1, 0, 0) blind 0.5 on bodies 3 bodies 3 in component "Breadboard"
extrude "Extrude12'" cut 2 faces at (-47.2093, 67.5, 3.3333) (-33.5427, 67.5, 3.3333) along direction (0, 1, 0) blind 0.5 on bodies 3 bodies 3 in component "Breadboard"
extrude "Extrude13'" cut 1 faces at (-35.376, 71, 3.3333) along direction (1, 0, 0) blind 0.5 on bodies 3 bodies 3 in component "Breadboard"
extrude "Extrude14'" cut 1 faces at (-45.376, 69.5, 3.3333) along direction (-1, 0, 0) blind 0.5 on bodies 3 bodies 3 in component "Breadboard"
extrude "Extrude15'" cut 3 faces at (11.9587, 72.5, 6.6667) (-54.7507, 72.5, 3.3333) (63.4587, 72.5, 6.6667) along direction (0, -1, 0) blind 0.5 on bodies 3 bodies 3 in component "Breadboard"
extrude "Extrude16'" cut 3 faces at (72.5, 54.2507, 6.6667) (72.5, -11.792, 3.3333) (72.5, -63.4587, 3.3333) along direction (-1, 0, 0) blind 0.5 on bodies 3 bodies 3 in component "Breadboard"
extrude "Extrude17'" cut 1 faces at (43.7093, 62.5, 3.3333) along direction (0, -1, 0) blind 0.5 on bodies 3 bodies 3 in component "Breadboard"
extrude "Extrude18'" cut 1 faces at (30.376, 63.8333, 6.6667) along direction (-1, 0, 0) blind 0.5 on bodies 3 bodies 3 in component "Breadboard"
extrude "Extrude19'" cut 1 faces at (50.376, 63.8333, 3.3333) along direction (1, 0, 0) blind 0.5 on bodies 3 bodies 3 in component "Breadboard"
extrude "Extrude20'" cut 2 faces at (31.7093, 67.5, 3.3333) (47.2093, 67.5, 3.3333) along direction (0, 1, 0) blind 0.5 on bodies 3 bodies 3 in component "Breadboard"
extrude "Extrude21'" cut 1 faces at (45.376, 70.6667, 3.3333) along direction (1, 0, 0) blind 0.5 on bodies 3 bodies 3 in component "Breadboard"
extrude "Extrude22'" cut 1 faces at (35.376, 69.3333, 3.3333) along direction (-1, 0, 0) blind 0.5 on bodies 3 bodies 3 in component "Breadboard"
extrude "Extrude23'" cut 1 faces at (62.5, 37.0427, 3.3333) along direction (-1, 0, 0) blind 0.5 on bodies 3 bodies 3 in component "Breadboard"
extrude "Extrude24'" cut 1 faces at (62.5, -43.7093, 3.3333) along direction (-1, 0, 0) blind 0.5 on bodies 3 bodies 3 in component "Breadboard"
extrude "Extrude25'" cut 4 faces at (67.5, 48.7093, 3.3333) (67.5, 32.0427, 6.6667) (67.5, -32.0427, 6.6667) (67.5, -48.7093, 3.3333) along direction (1, 0, 0) blind 0.5 on bodies 3 bodies 3 in component "Breadboard"
extrude "Extrude26'" cut 1 faces at (64, 50.376, 3.3333) along direction (0, 1, 0) blind 0.5 on bodies 3 bodies 3 in component "Breadboard"
extrude "Extrude27'" cut 1 faces at (66, 30.376, 3.3333) along direction (0, -1, 0) blind 0.5 on bodies 3 bodies 3 in component "Breadboard"
extrude "Extrude28'" cut 1 faces at (69.3333, 35.376, 3.3333) along direction (0, -1, 0) blind 0.5 on bodies 3 bodies 3 in component "Breadboard"
extrude "Extrude29'" cut 1 faces at (70.6667, 45.376, 3.3333) along direction (0, 1, 0) blind 0.5 on bodies 3 bodies 3 in component "Breadboard"
extrude "Extrude30'" cut 1 faces at (69.3333, -35.376, 3.3333) along direction (0, 1, 0) blind 0.5 on bodies 3 bodies 3 in component "Breadboard"
extrude "Extrude31'" cut 1 faces at (70.6667, -45.376, 3.3333) along direction (0, -1, 0) blind 0.5 on bodies 3 bodies 3 in component "Breadboard"
extrude "Extrude32'" cut 1 faces at (66, -50.376, 3.3333) along direction (0, -1, 0) blind 0.5 on bodies 3 bodies 3 in component "Breadboard"
extrude "Extrude33'" cut 1 faces at (64, -30.376, 3.3333) along direction (0, 1, 0) blind 0.5 on bodies 3 bodies 3 in component "Breadboard"